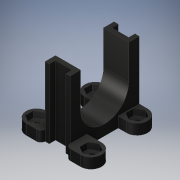
# Autodesk Inventor part: SupportBatterie
Saved by Autodesk Inventor 2019 (Build 230136000, 136)
## iProperties
Created: 2019-07-30
Part Number: SupportBatterie
Material: Plastique ABS
Document SubType Name: Modeling
Designer: Sébastien DI MERCURIO
Mass: 42.8155 g
Surface Area: 70.68 cm^2
Volume: 40.392 cm^3
Density: 1.06 g/cm^3
Appearance: Lustré - Noir
Author: Sébastien DI MERCURIO
Autodesk Inventor part; units mm, degrees
ref_plane "XZ Plane" through (0, 0, 0) normal (0, 1, 0) x (-1, 0, 0)
ref_plane "XY Plane" through (0, 0, 0) normal (0, 0, 1) x (1, 0, 0)
sketch "Esquisse2" plane through (0, 0, 0) normal (0, 1, 0) x (-1, 0, 0)
  line L0 (0, 0) -> (36, 0)
  line L1 (36, 0) -> (36, -35)
  line L2 (36, -35) -> (0, -35)
  line L3 (0, -35) -> (0, 0)
  dimension "d0" = 35
  dimension "d1" = 36
  constraints: 8 end point, 2 parallel, 1 horizontal, 1 perpendicular
  measures "d0" distance of L0.end L1.end
  measures "d1" distance of L1.end L2.end
extrude "Extrusion1" add sketch "Esquisse2" along normal blind 33
sketch "Esquisse3" plane through (0, 33, 0) normal (0, 1, 0) x (1, 0, 0)
  line L0 (0, 35) -> (-36, 35) projected
  line L1 (0, 0) -> (-12, 0)
  line L2 (-12, 0) -> (-12, 35)
  line L3 (-12, 35) -> (0, 35)
  line L4 (0, 35) -> (0, 0)
  line L5 (-36, 0) -> (0, 0) projected
  line L6 (-36, 0) -> (-24, 0)
  line L7 (-24, 0) -> (-24, 35)
  line L8 (-24, 35) -> (-36, 35)
  line L9 (-36, 35) -> (-36, 0)
  dimension "d4" = 12
  dimension "d5" = 12
  constraints: 16 end point, 4 parallel, 2 horizontal, 2 perpendicular, 2 point on line
  measures "d4" distance between parallel lines of L7 L9
  measures "d5" distance between parallel lines of L4 L2
extrude "Extrusion2" cut sketch "Esquisse3" against normal blind 28 contours L4 L1 L2 L0 | L7 L5 L9 L0
sketch "Esquisse4" plane through (0, 33, 0) normal (0, 1, 0) x (1, 0, 0)
  line L0 (-24, 0) -> (-12, 0) projected
  line L1 (-24, 0) -> (-12, 0)
  line L2 (-12, 0) -> (-12, 2)
  line L3 (-24, 2) -> (-24, 0)
  line L4 (-14, 2) -> (-14, 5)
  line L5 (-14, 5) -> (-22, 5)
  line L6 (-22, 5) -> (-22, 2)
  line L7 (-12, 35) -> (-24, 35) projected
  line L8 (-22, 35) -> (-14, 35)
  line L9 (-14, 35) -> (-14, 32)
  line L10 (-14, 32) -> (-22, 32)
  line L11 (-22, 32) -> (-22, 35)
  line L12 (-12, 0) -> (-12, 35) projected
  line L13 (-24, 35) -> (-24, 0) projected
  line L14 (-14, 2) -> (-12, 2)
  line L15 (-24, 2) -> (-22, 2)
  point P0 (0, 0)
  dimension "d8" = 3
  dimension "d11" = 8
  dimension "d12" = 12
  dimension "d14" = 2
  dimension "d15" = 2
  constraints: 24 end point, 4 collinear, 4 parallel, 4 point on line, 3 perpendicular, 2 horizontal
  measures "d8" distance of L10.end L8.start
  measures "d11" distance between parallel lines of L4 L6
  measures "d12" distance between parallel lines of L12 L13
  measures "d14" distance of L3.start L6.end
  measures "d15" distance between parallel lines of L0 L15
extrude "Extrusion3" cut sketch "Esquisse4" against normal through all contours L3 L15 L6 L5 L4 L14 L2 L0 | L7 L9 L10 L11
sketch "Esquisse5" plane through (-12, 5, -35) normal (1, 0, 0) x (0, 0, -1)
  line L0 (-16.5, 11.5) -> (-16.5, 94.3669) construction
  line L1 (-5, 11.5) -> (-5, 94.3669)
  line L2 (-28, 94.3669) -> (-28, 11.5)
  arc A0 (-28, 11.5) -> (-5, 11.5) centre (-16.5, 11.5) ccw
  arc A1 (-5, 94.3669) -> (-28, 94.3669) centre (-16.5, 94.3669) ccw
  line L3 (0, 28) -> (0, 0) projected
  line L4 (0, -5) -> (-35, -5) projected
  point P0 (-16.5, 52.9334)
  dimension "d18" = 23
  dimension "d19" = 5
  dimension "d20" = 5
  constraints: 8 end point, 4 point on circle, 4 tangent, 2 centre point, 1 midpoint, 1 parallel, 1 vertical
  measures "d18" distance between parallel lines of L1 L2
  measures "d19" distance between parallel lines of L3 L1
  measures "d20" distance edge to line of A0 L4
extrude "Extrusion4" cut sketch "Esquisse5" against normal through all
sketch "Esquisse6" plane through (0, 5, 0) normal (0, 1, 0) x (1, 0, 0)
  line L0 (-36, 0) -> (-36, 35) projected
  line L1 (-36, 10) -> (-36, 35)
  line L2 (-36, 35) -> (-33, 35)
  line L3 (-33, 35) -> (-33, 25)
  line L4 (-33, 25) -> (-24, 25)
  line L5 (-24, 35) -> (-24, 18.5) projected
  line L6 (-24, 18.5) -> (-24, 2) projected
  line L7 (-24, 10) -> (-36, 10)
  line L8 (-24, 0) -> (-36, 0) projected
  line L9 (-36, 35) -> (-24, 35) projected
  line L10 (-18, -7.1918) -> (-18, 53.3139) construction
  point P0 (0, 0)
  dimension "d23" = 10
  dimension "d24" = 10
  dimension "d25" = 3
  dimension "d26" = 36
  dimension "d27" = 18
  constraints: 12 end point, 4 perpendicular, 3 point on line, 1 collinear, 1 vertical
  measures "d23" distance between parallel lines of L8 L7
  measures "d24" distance between parallel lines of L9 L4
  measures "d25" distance of L2.end L0.end
  measures "d26" distance of point (0, 0) L0.start
  measures "d27" distance from line of L10 L0.start
extrude "Extrusion5" cut sketch "Esquisse6" against normal through all contours L0 L2 L3 L4 L5 L6 L7
ref_plane "Plan de construction1" through (-18, 0, 0) normal (1, 0, 0) x (0, 1, 0)
mirror "Symétrie1" about plane through (-18, 0, 0) normal (1, 0, 0) of "Extrusion5"
sketch "Esquisse8" plane through (0, 5, 0) normal (0, 1, 0) x (1, 0, 0)
  circle A0 centre (-31, 5) radius 1.5
  circle A1 centre (-28, 30) radius 1.5
  line L0 (-24, 10) -> (-36, 10) projected
  line L1 (-24, 0) -> (-36, 0) projected
  line L2 (-33, 35) -> (-24, 35) projected
  line L3 (-33, 25) -> (-24, 25) projected
  line L4 (-18, 42) -> (-18, -7) projected
  point P0 (0, 0)
  dimension "d31" = 3
  dimension "d32" = 10
  dimension "d33" = 5
  dimension "d34" = 10
  dimension "d35" = 5
  dimension "d36" = 13
  dimension "d37" = 10
  constraints: 2 centre point, 1 equal radius
  measures "d31" diameter of A0
  measures "d32" distance between parallel lines of L0 L1
  measures "d33" distance from line of L1 A0.centre
  measures "d34" distance between parallel lines of L2 L3
  measures "d35" distance from line of L3 A1.centre
  measures "d36" distance from line of A0.centre L4
  measures "d37" distance from line of L4 A1.centre
extrude "Extrusion6" cut sketch "Esquisse8" against normal through all
sketch "Esquisse9" plane through (0, 5, 0) normal (0, 1, 0) x (1, 0, 0)
  circle A0 centre (-31, 5) radius 1.5 projected
  line L0 (-31, 0.9585) -> (-34.5, 2.9793)
  line L1 (-34.5, 2.9793) -> (-34.5, 7.0207)
  line L2 (-34.5, 7.0207) -> (-31, 9.0415)
  line L3 (-31, 9.0415) -> (-27.5, 7.0207)
  line L4 (-27.5, 7.0207) -> (-27.5, 2.9793)
  line L5 (-27.5, 2.9793) -> (-31, 0.9585)
  circle A1 centre (-28, 30) radius 1.5 projected
  line L6 (-28, 25.9585) -> (-31.5, 27.9793)
  line L7 (-31.5, 27.9793) -> (-31.5, 32.0207)
  line L8 (-31.5, 32.0207) -> (-28, 34.0415)
  line L9 (-28, 34.0415) -> (-24.5, 32.0207)
  line L10 (-24.5, 32.0207) -> (-24.5, 27.9793)
  line L11 (-24.5, 27.9793) -> (-28, 25.9585)
  point P0 (0, 0)
  dimension "d40" = 7
  constraints: 24 end point, 2 coincident, 2 vertical alignment, 1 parallel, 26 other
  measures "d40" distance between parallel lines of L1 L4
extrude "Extrusion7" cut sketch "Esquisse9" against normal blind 3
fillet "Congé1" radius 5 4 edges at (-36, 2.5, 0) (-36, 2.5, -10) (-33, 2.5, -25) (-33, 2.5, -35)
fillet "Congé2" radius 2 1 edges at (-24, 2.5, 0)
mirror "Symétrie2" about plane through (-18, 0, 0) normal (1, 0, 0) of "Extrusion6", "Extrusion7", "Congé1", "Congé2"
equation "\"d5\" = d4"
equation "\"d14\" = -0.5 * d11 + 0.5 * d12"
equation "\"d27\" = 0.5 * d26"
equation "\"d33\" = 0.5 * d32"
equation "\"d35\" = 0.5 * d34"
